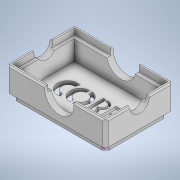
# Autodesk Inventor part: rack holder aliminium 2
Saved by Autodesk Inventor 2021 (Build 250183000, 183)
## iProperties
Created: 2021-05-21
Part Number: rack holder aliminium 2
Material: Generic
Document SubType Name: Modeling
Designer: Olivi
Density: 1 g/cm^3
Appearance: Default
Author: Olivi
Autodesk Inventor part; units mm, degrees
ref_plane "YZ Plane" through (0, 0, 0) normal (1, 0, 0) x (0, 1, 0)
ref_plane "XZ Plane" through (0, 0, 0) normal (0, 1, 0) x (-1, 0, 0)
ref_plane "XY Plane" through (0, 0, 0) normal (0, 0, 1) x (1, 0, 0)
sketch "Sketch1" plane through (0, 0, 0) normal (0, 1, 0) x (-1, 0, 0)
  line L0 (0, 0) -> (0, -86)
  line L1 (0, -86) -> (128.3, -86)
  line L2 (128.3, -86) -> (128.3, 0)
  line L3 (128.3, 0) -> (0, 0)
  dimension "d0" = 86
  dimension "d1" = 128.3
  constraints: 8 end point, 3 perpendicular, 1 vertical
  measures "d0" distance of L0.start L0.end
  measures "d1" distance of L0.end L1.end
extrude "Extrusion2" add sketch "Sketch1" along normal blind 6
sketch "Sketch3" plane through (0, 6, 0) normal (0, 1, 0) x (1, 0, 0)
  point P0 (0, 0)
sketch "Sketch4" plane through (0, 6, 0) normal (0, 1, 0) x (1, 0, 0)
  arc A0 (-91.2531, 56.696) -> (-91.5743, 29.7143) centre (-95.2962, 43.2514) ccw
  arc A1 (-93.1804, 51.2354) -> (-93.1804, 34.2112) centre (-94.0166, 42.7233) ccw
  line L0 (-93.1804, 51.2354) -> (-91.2531, 56.696)
  line L1 (-93.1804, 34.2112) -> (-91.5743, 29.7143)
  arc A2 (-78.0632, 52.0407) -> (-78.3199, 34.448) centre (-76.5372, 43.2202) ccw
  arc A3 (-74.7545, 34.448) -> (-75.0113, 52.0407) centre (-76.5372, 43.2202) ccw
  arc A4 (-75.0113, 29.7143) -> (-75.0113, 56.696) centre (-76.1328, 43.2051) ccw
  line L2 (-75.0113, 56.696) -> (-75.0113, 52.0407)
  line L3 (-74.7545, 34.448) -> (-75.0113, 29.7143)
  line L4 (-78.3199, 34.448) -> (-78.3199, 29.4603)
  line L5 (-78.0632, 56.6961) -> (-78.0632, 52.0407)
  arc A5 (-78.0632, 56.6961) -> (-78.3199, 29.4603) centre (-77.9302, 43.0757) ccw
  line L6 (-59.5494, 56.6961) -> (-59.5494, 29.4603)
  line L7 (-59.5494, 29.4603) -> (-55.5494, 29.4603)
  line L8 (-55.5494, 29.4603) -> (-55.5494, 56.6961)
  line L9 (-55.5494, 56.6961) -> (-59.5494, 56.6961)
  line L10 (-47.4135, 29.4603) -> (-53.7861, 43.0782)
  arc A6 (-53.7861, 43.0782) -> (-53.7861, 54.3684) centre (-53.0876, 48.7233) ccw
  line L11 (-47.4135, 29.4603) -> (-43.9803, 31.0669)
  line L12 (-43.9803, 31.0669) -> (-48.5954, 40.9288)
  arc A7 (-48.5954, 40.9288) -> (-53.7861, 56.6961) centre (-52.5494, 48.3652) ccw
  line L13 (-53.7861, 56.6961) -> (-53.7861, 54.3684)
  line L14 (-41.5494, 56.0046) -> (-41.5494, 29.4603)
  line L15 (-41.5494, 29.4603) -> (-27.5494, 29.4603)
  line L16 (-27.5494, 29.4603) -> (-27.5494, 33.1666)
  line L17 (-27.5494, 33.1666) -> (-37.5494, 33.1666)
  line L18 (-37.5494, 33.1666) -> (-37.5494, 41.4179)
  line L19 (-37.5494, 41.4179) -> (-29.2175, 41.4179)
  line L20 (-29.2175, 41.4179) -> (-29.2175, 44.4179)
  line L21 (-29.2175, 44.4179) -> (-37.5494, 44.4179)
  line L22 (-37.5494, 44.4179) -> (-37.5494, 52.4179)
  line L23 (-37.5494, 52.4179) -> (-27.5494, 52.4179)
  line L24 (-27.5494, 52.4179) -> (-27.5494, 56.0046)
  line L25 (-27.5494, 56.0046) -> (-41.5494, 56.0046)
  line L26 (-128.3, 86) -> (-128.3, 0) projected
  line L27 (0, 86) -> (-128.3, 86) projected
  point P0 (0, 0)
  constraints: 52 end point, 19 point on circle, 13 perpendicular, 8 centre point, 6 vertical, 5 point on line, 1 concentric
extrude "Extrusion3" cut sketch "Sketch4" against normal through all
sketch "Sketch26" plane through (0, 6, 0) normal (0, 1, 0) x (1, 0, 0)
  point P0 (0, 0)
sketch "Sketch27" plane through (0, 6, 0) normal (0, 1, 0) x (1, 0, 0)
  line L0 (-1.7618, -2.4025) -> (1.922, -2.4025)
  point P0 (0, 0)
  constraints: 2 end point, 1 horizontal
sketch "Sketch28" plane through (0, 6, 0) normal (0, 1, 0) x (1, 0, 0)
  point P0 (0, 0)
sketch "Sketch29" plane through (0, 6, 0) normal (0, 1, 0) x (1, 0, 0)
  line L0 (0, 86) -> (-128.3, 86) projected
  line L1 (-128.3, 86) -> (0, 86)
  line L2 (-128.3, 0) -> (0, 0) projected
  line L3 (0, 86) -> (0, 0)
  line L4 (0, 0) -> (-128.3, 0)
  line L5 (-128.3, 0) -> (-128.3, 86)
  line L6 (-132.3, -4) -> (-132.3, 90)
  line L7 (-132.3, 90) -> (4, 90)
  line L8 (4, 90) -> (4, -4)
  line L9 (4, -4) -> (-132.3, -4)
  dimension "d114" = 4
  dimension "d115" = 4
  dimension "d116" = 4
  dimension "d117" = 4
  constraints: 16 end point, 4 perpendicular, 2 collinear, 1 parallel, 1 vertical
  measures "d114" distance between parallel lines of L0 L7
  measures "d115" distance between parallel lines of L8 L3
  measures "d116" distance between parallel lines of L5 L6
  measures "d117" distance between parallel lines of L9 L2
extrude "Extrusion11" add sketch "Sketch29" along normal blind 35 and the other way blind 6
sketch "Sketch30" plane through (-132.3, 41, 4) normal (0, 0, 1) x (1, 0, 0)
  line L0 (4, 0) -> (132.3, 0) projected
  arc A0 (53.4147, 0) -> (92.5853, 0) centre (73, -4.0519) ccw
  line L1 (53.4147, 0) -> (92.5853, 0)
  line L2 (0, -41) -> (0, 0) projected
  point P0 (132.3, -41)
  dimension "d160" = 20
  dimension "d161" = 73
  constraints: 2 end point, 2 point on circle, 2 point on line, 1 centre point, 1 collinear
  measures "d160" radius of A0
  measures "d161" distance from line of A0.centre L2
extrude "Extrusion12" cut sketch "Sketch30" against normal through all
chamfer "Chamfer1" distance 4 angle 45 2 edges at (4, 20.5, 4) (4, 20.5, -90)
chamfer "Chamfer2" distance 4 angle 45 2 edges at (-132.3, 20.5, 4) (-132.3, 20.5, -90)
sketch "Sketch41" plane through (0, 6, 0) normal (0, 1, 0) x (1, 0, 0)
  line L0 (-123.8, 4.6) -> (-4.5, 4.6)
  line L1 (0, 0) -> (0, 86) projected
  line L2 (-123.8, 4.6) -> (-123.8, 80.8)
  line L3 (-123.8, 80.8) -> (-4.5, 80.8)
  line L4 (-4.5, 80.8) -> (-4.5, 4.6)
  line L5 (-128.3, 55.5427) -> (-128.3, 30.4573) projected
  line L6 (-79.3, 0) -> (-39.3, 0) projected
  line L7 (-128.3, 0) -> (0, 0) projected
  line L8 (0, 0) -> (-128.3, 0)
  line L9 (0, 86) -> (-128.3, 86) projected
  line L10 (-128.3, 0) -> (-128.3, 86)
  line L11 (-128.3, 86) -> (0, 86)
  line L12 (0, 86) -> (0, 0)
  point P0 (-128.3, 55.5)
  point P1 (-128.3, 30.5)
  point P2 (-78.8853, 0)
  point P3 (-39.7147, 0)
  dimension "d188" = 119.3
  dimension "d189" = 4.5
  dimension "d190" = 4.6
  dimension "d191" = 76.2
  constraints: 16 end point, 4 perpendicular, 2 collinear, 1 horizontal, 1 vertical
  measures "d188" distance of L0.start L0.end
  measures "d189" distance between parallel lines of L5 L2
  measures "d190" distance between parallel lines of L6 L0
  measures "d191" distance of L3.end L0.end
extrude "Extrusion22" add sketch "Sketch41" along normal blind 26.6
sketch "Sketch42" plane through (-59.3, 36.9481, 4) normal (0, 0, 1) x (1, 0, 0)
  line L0 (-27.5, 4.0519) -> (100.8, 4.0519)
  arc A0 (-19.5853, 4.0519) -> (19.5853, 4.0519) centre (0, 0) ccw
  line L1 (-19.5853, 4.0519) -> (19.5853, 4.0519)
  line L2 (0, 27.822) -> (0, 103.4366)
  line L3 (19.5853, 4.0519) -> (59.3, 4.0519) projected
  arc A1 (-19.5853, 4.0519) -> (19.5853, 4.0519) centre (0, 0) ccw projected
  point P0 (59.3, -36.9481)
  point P1 (137.3, -41)
  dimension "d194" = 20
  dimension "d195" = 0
  dimension "d196" = 0
  dimension "d197" = 0
  dimension "d198" = 0
  constraints: 6 end point, 2 point on circle, 2 point on line, 1 centre point, 1 collinear
  measures "d194" radius of A0
  measures "d195" distance from line of A0.centre L2
  measures "d196" horizontal distance of L2.end A0.centre
  measures "d197" distance between parallel lines of L3 L0
  measures "d198" distance of A1.centre A0.centre
extrude "Extrusion23" cut sketch "Sketch42" against normal through all
sketch "Sketch45" plane through (4, 0, -86) normal (1, 0, 0) x (0, 0, -1)
  line L0 (0, 41) -> (-86, 41) projected
  arc A0 (-56.2832, 41) -> (-29.7168, 41) centre (-43, 40.0517) ccw
  line L1 (-56.2832, 41) -> (-29.7168, 41)
  line L2 (-86, 0) -> (-86, 41) projected
  arc A1 (-59.2337, 41) -> (-36.4934, 41) centre (-47.8635, 40.569) ccw
  line L3 (-59.2337, 41) -> (-36.4934, 41)
  point P0 (-86, 0)
  dimension "d204" = 43
  constraints: 4 end point, 4 point on circle, 4 point on line, 2 centre point, 1 collinear, 1 horizontal
  measures "d204" distance from line of L2 A0.centre
extrude "Extrusion24" cut sketch "Sketch45" against normal through all contours A0 A1 L0 | A1 A0 L0 picked at (-32.0225, 39.9683) picked at (-50.0029, 38.1705)
sketch "Sketch46" plane through (0, 0, 0) normal (0, -1, 0) x (1, 0, 0)
  line L0 (-137.3, 18.3069) -> (-137.3, -100.8343)
  line L1 (-137.3, -100.8343) -> (10.6494, -100.8343)
  line L2 (10.6494, -100.8343) -> (10.6494, 18.3069)
  line L3 (10.6494, 18.3069) -> (-137.3, 18.3069)
  line L4 (0, -31.9631) -> (0, 0) projected
  line L5 (0, 0) -> (0, -85.5)
  line L6 (0, -86) -> (0, 0) projected
  line L7 (-128.3, -86) -> (-78.8853, -86) projected
  line L8 (0, 0) -> (-39.7784, 0) projected
  line L9 (0, 0) -> (-127.7, 0)
  line L10 (-128.3, 0) -> (-128.3, -29.7168) projected
  line L11 (-127.7, 0) -> (-127.7, -85.5)
  line L12 (-127.7, -85.5) -> (0, -85.5)
  point P0 (0, -30.0148)
  point P1 (0, -46.2581)
  point P2 (-128.3, -26.7663)
  point P3 (0, -30.0148)
  dimension "d214" = 85.5
  dimension "d216" = 127.7
  constraints: 16 end point, 5 perpendicular, 1 point on line, 1 vertical
  measures "d214" distance of L4.end L5.end
  measures "d216" distance of L4.end L9.end
extrude "Extrusion25" cut sketch "Sketch46" against normal blind 8
chamfer "Chamfer3" distance 5 angle 45 4 edges at (0, 4, 0) (0, 4, -85.5) (-127.7, 4, 0) (-127.7, 4, -85.5)
chamfer "Chamfer5" distance 2 angle 45 8 edges at (4, 41, -14.8584) (-19.8574, 41, 4) (-103.5926, 41, 4) (-132.3, 41, -14.8584) (-132.3, 41, -71.1416) (-103.5926, 41, -90) (-19.8574, 41, -90) (4, 41, -71.1416)
body "Solid2"
